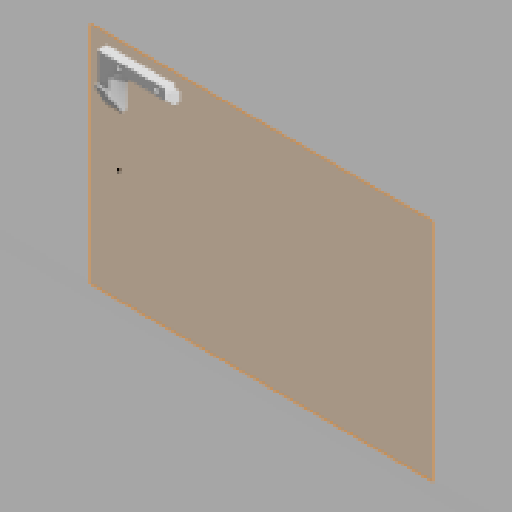
# Autodesk Inventor part: Накладка_левая
Saved by Autodesk Inventor 2025 (Build 290162000, 162)
## iProperties
Created: 2025-04-24
Part Number: Накладка_левая
Material: Типовые
Document SubType Name: Modeling
Designer: Artem Sannikov
Density: 1 g/cm^3
Appearance: По умолчанию
Author: Artem Sannikov
Autodesk Inventor part; units mm, degrees
ref_plane "YZ Plane" through (0, 0, 0) normal (1, 0, 0) x (0, 1, 0)
ref_plane "XZ Plane" through (0, 0, 0) normal (0, 1, 0) x (-1, 0, 0)
ref_plane "РабПлоскость1" through (0, 0, 0) normal (0, 0, 1) x (1, 0, 0)
sketch "Эскиз1" plane through (0, 0, 0) normal (0, 0, 1) x (1, 0, 0)
  line L0 (265, 175) -> (-265, 175)
  line L1 (-265, 175) -> (-265, -175)
  line L2 (-265, 125) -> (-245, 125)
  line L3 (-245, 125) -> (-245, 143)
  line L4 (-245, 143) -> (-230, 158)
  line L5 (-230, 158) -> (-149.3726, 158)
  line L6 (-149.3726, 158) -> (-149.3726, 178)
  point P0 (0, 0)
  point P1 (-149.3726, 175)
extrude "Выдавливание1" add sketch "Эскиз1" along normal blind 15.7
sketch "Эскиз2" plane through (-245, 125, 0) normal (1, 0, 0) x (0, 0, -1)
  line L0 (0, 0) -> (-15.7, 0) projected
  line L1 (-20, -4) -> (0, -38.641) projected
  line L2 (-20, -4) -> (-20, 0) projected
  line L3 (0, 50) -> (0, -300) projected
  line L4 (-20, 0) -> (-15.7574, 0) projected
  line L5 (-20, 0) -> (0, 0)
  line L6 (0, -38.641) -> (0, 0)
  point P0 (0, -125)
  point P1 (-15.7574, 0)
  constraints: 4 end point, 1 collinear, 1 horizontal
ref_plane "РабПлоскость2" through (-265, -125, -86) normal (1, 0, 0) x (0, 1, 0)
extrude "Выдавливание2" add sketch "Эскиз2" against normal up to surface (20 mm away)
sketch "Эскиз3" plane through (-230, 158, 0) normal (0, -1, 0) x (1, 0, 0)
  line L0 (91.2262, -0.185) -> (79.9532, 15.7574) projected
  line L1 (80.6274, 0) -> (80.6274, 15.7) projected
  line L2 (0, 0) -> (80.6274, 0) projected
  line L3 (80.6274, 0) -> (91.2262, -0.185)
  point P0 (230, 0)
  point P1 (80.6274, 14.8038)
  constraints: 2 end point
extrude "Выдавливание3" add sketch "Эскиз3" against normal blind 10.75
sketch "Эскиз4" plane through (0, 0, 0) normal (0, 0, -1) x (-1, 0, 0)
  line L0 (245, 143) -> (230, 158) projected
  line L1 (230, 158) -> (149.3726, 158) projected
  line L2 (245, 86.359) -> (245, 143) projected
  line L3 (149.3726, 158) -> (138.7738, 158) projected
  line L4 (148.7738, 143) -> (149.3726, 143)
  line L5 (149.3726, 143) -> (223.7868, 143)
  line L6 (223.7868, 143) -> (230, 136.7868)
  line L7 (230, 136.7868) -> (230, 96.359)
  line L8 (138.7738, 153) -> (138.7738, 158)
  line L9 (240, 86.359) -> (245, 86.359)
  line L10 (240, 86.359) -> (230, 96.359)
  line L11 (148.7738, 143) -> (138.7738, 153)
  point P0 (0, 0)
  point P1 (138.7738, 143)
  point P2 (230, 86.359)
  dimension "d6" = 15
  dimension "d7" = 10
  dimension "d8" = 10
  dimension "d9" = 10
  dimension "d10" = 10
  constraints: 16 end point, 4 point on line, 1 perpendicular, 1 vertical, 3 other
  measures "d6" distance between parallel lines of L0 L6
  measures "d7" distance of L9.start point (230, 86.359)
  measures "d8" distance of L7.end point (230, 86.359)
  measures "d9" distance of L4.start point (138.774, 143)
  measures "d10" distance of L8.start point (138.774, 143)
extrude "Выдавливание4" add sketch "Эскиз4" against normal blind 1
chamfer "Фаска1" distance 14.5 angle 45 3 edges at (-237.5, 150.5, 1) (-184.8059, 158, 1) (-245, 115.5455, 1)
sketch "Эскиз5" plane through (-245, 86.359, 15.5) normal (-1, 0, 0) x (0, 0, 1)
  point P0 (-15.5, -86.359)
sketch "Эскиз6" plane through (-245, 86.359, 15.5) normal (-1, 0, 0) x (0, 0, 1)
  line L0 (0, 26.8468) -> (-15.5, 0) projected
  line L1 (-15.5, 0) -> (0, 0) projected
  line L2 (0, 26.8468) -> (0, 0) projected
  point P0 (-15.5, -86.359)
extrude "Выдавливание5" cut sketch "Эскиз6" against normal blind 19.5
sketch "Эскиз7" plane through (-149.3726, 158, 15.5) normal (0, 1, 0) x (1, 0, 0)
  line L0 (10.4679, 15.5) -> (0, 0.6962) projected
  line L1 (0, 0.6962) -> (0, 0) projected
  line L2 (0, 0) -> (10.5987, 0) projected
  line L3 (10.5987, 15.5) -> (10.5987, 0) projected
  line L4 (10.4679, 15.5) -> (10.5987, 15.5) projected
  point P0 (149.3726, 15.5)
extrude "Выдавливание6" cut sketch "Эскиз7" against normal blind 19.5
sketch "Эскиз8" plane through (0, 0, 15.7) normal (0, 0, 1) x (1, 0, 0)
  circle A0 centre (-164.3726, 165) radius 3.25 projected
  circle A1 centre (-228.3726, 165) radius 3.25 projected
  point P0 (0, 0)
extrude "Выдавливание7" cut sketch "Эскиз8" against normal blind 28.75
equation "\"d8\" = d7"
equation "\"d9\" = d7"
equation "\"d10\" = d9"
